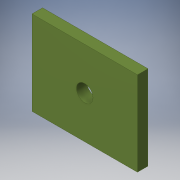
# Autodesk Inventor part: 2 x 2_5 x 1_4
Saved by Autodesk Inventor 2016 (Build 200138000, 138)
## iProperties
Created: 2015-06-19
Part Number: 2 x 2_5 x 1_4
Material: Aluminum 6061
Document SubType Name: Modeling
Designer: steele
Density: 2.7 g/cm^3
Appearance: Dark Olive
Mass: 65.0121 g
Surface Area: 93.9685 cm^2
Volume: 24.0786 cm^3
Author: steele
Autodesk Inventor part; units mm, degrees
ref_plane "YZ Plane" through (0, 0, 0) normal (1, 0, 0) x (0, 1, 0)
ref_plane "XZ Plane" through (0, 0, 0) normal (0, 1, 0) x (-1, 0, 0)
ref_plane "XY Plane" through (0, 0, 0) normal (0, 0, 1) x (1, 0, 0)
sketch "Sketch1" plane through (0, 0, 0) normal (0, 0, 1) x (1, 0, 0)
  line L0 (-31.75, -25.4) -> (31.75, -25.4)
  line L1 (31.75, -25.4) -> (31.75, 25.4)
  line L2 (31.75, 25.4) -> (-31.75, 25.4)
  line L3 (-31.75, 25.4) -> (-31.75, -25.4)
  line L4 (-31.75, -25.4) -> (31.75, 25.4) construction
  line L5 (31.75, -25.4) -> (-31.75, 25.4) construction
  point P0 (0, 0)
  dimension "height" = 50.8
  dimension "width" = 63.5
  constraints: 12 end point, 2 midpoint, 2 parallel, 1 horizontal, 1 perpendicular
  measures "height" distance of L1.end L0.end
  measures "width" distance of L1.end L2.end
extrude "Extrusion1" add sketch "Sketch1" along normal mid plane 6.35
sketch "Sketch2" plane through (0, 0, 3.175) normal (0, 0, 1) x (1, 0, 0)
  line L0 (31.75, 25.4) -> (-31.75, 25.4) construction
  line L1 (0, 25.4) -> (0, -25.4) construction
  line L2 (-31.75, -25.4) -> (31.75, -25.4) construction
  line L3 (-38.1, 0) -> (31.75, 0) construction
  line L4 (31.75, -25.4) -> (31.75, 25.4) construction
  circle A0 centre (0, 0) radius 5.0165
  dimension "heightOfHole" = 25.4
  dimension "holeDiameter" = 10.033
  constraints: 4 end point, 3 midpoint, 1 centre point, 1 coincident, 1 horizontal
  measures "heightOfHole" distance between parallel lines of L2 L3
  measures "holeDiameter" diameter of A0
extrude "Extrusion3" cut sketch "Sketch2" against normal through all
body "Solid1"
